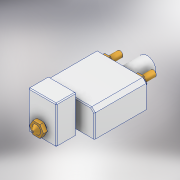
# Autodesk Inventor part: Arethusa
Saved by Autodesk Inventor 2022.1 (Build 261234020, 234B)
## iProperties
Created: 2022-04-17
Part Number: Arethusa
Material: Aluminum 6061
Document SubType Name: Modeling
Designer: Remo
Density: 2.7 g/cm^3
Appearance: Aluminum - Flat
Author: Remo
Autodesk Inventor part; units mm, degrees
ref_plane "YZ Plane" through (0, 0, 0) normal (1, 0, 0) x (0, 1, 0)
ref_plane "XZ Plane" through (0, 0, 0) normal (0, 1, 0) x (-1, 0, 0)
ref_plane "XY Plane" through (0, 0, 0) normal (0, 0, 1) x (1, 0, 0)
sketch "Sketch1" plane through (0, 0, 0) normal (0, 0, 1) x (1, 0, 0)
  line L0 (15, -7.5) -> (-15, -7.5)
  line L1 (-15, -7.5) -> (-15, 7.5)
  line L2 (-15, 7.5) -> (15, 7.5)
  line L3 (15, 7.5) -> (15, -7.5)
  line L4 (15, -7.5) -> (-15, 7.5) construction
  line L5 (-15, -7.5) -> (15, 7.5) construction
  point P0 (0, 0)
  dimension "d0" = 15
  dimension "d1" = 30
  constraints: 12 end point, 2 midpoint, 2 parallel, 1 horizontal, 1 perpendicular
  measures "d0" distance of L0.end L1.end
  measures "d1" distance of L1.end L2.end
extrude "Extrusion1" add sketch "Sketch1" along normal blind 30
sketch "Sketch2" plane through (0, 0, 30) normal (0, 0, 1) x (1, 0, 0)
  line L0 (15, 7.5) -> (-15, 7.5) projected
  line L1 (-15, 7.5) -> (-15, -7.5) projected
  line L2 (-15, -7.5) -> (15, -7.5) projected
  line L3 (15, -7.5) -> (15, 7.5) projected
  circle A0 centre (0, -1) radius 2.5
  point P0 (0, 0)
  dimension "d4" = 6.5
  dimension "d5" = 5
  constraints: 1 centre point, 1 vertical alignment
  measures "d4" distance from line of L2 A0.centre
  measures "d5" diameter of A0
extrude "Extrusion2" add sketch "Sketch2" along normal blind 3.3 contours A0
sketch "Sketch3" plane through (0, -1, 33.3) normal (0, 0, 1) x (1, 0, 0)
  circle A0 centre (0, 0) radius 2.5 projected
  line L0 (-8, 15) -> (8, 15)
  line L1 (8, 15) -> (8, -8)
  line L2 (8, -8) -> (-8, -8)
  line L3 (-8, -8) -> (-8, 15)
  line L4 (-8, 15) -> (8, -8) construction
  line L5 (8, 15) -> (-8, -8) construction
  line L6 (-15, -6.5) -> (15, -6.5) projected
  point P0 (0, 1)
  point P1 (0, 3.5)
  point P2 (0, 3.5)
  point P3 (-8, -6.5)
  point P4 (8, -6.5)
  dimension "d9" = 23
  dimension "d10" = 16
  dimension "d11" = 8
  constraints: 12 end point, 3 midpoint, 2 parallel, 1 horizontal, 1 perpendicular, 1 vertical alignment
  measures "d9" distance of L2.end L0.start
  measures "d10" distance of L0.start L0.end
  measures "d11" distance from line of L2 A0.centre
extrude "Extrusion3" add sketch "Sketch3" along normal blind 11.5 contours A0 | L0 L1 L6 L3
sketch "Sketch4" plane through (-15, -7.5, 0) normal (0, -1, 0) x (1, 0, 0)
  line L0 (0, 0) -> (30, 0) projected
  line L1 (30, 0) -> (30, 30) projected
  line L2 (0, 30) -> (30, 30) projected
  line L3 (0, 0) -> (0, 30) projected
  circle A0 centre (7, 7) radius 1.4
  circle A1 centre (23, 7) radius 1.4
  circle A2 centre (7, 23) radius 1.4
  circle A3 centre (23, 23) radius 1.4
  point P0 (15, 0)
  point P1 (15, 30)
  dimension "d16" = 16
  dimension "d19" = 16
  dimension "d22" = 8
  dimension "d23" = 7
  dimension "d24" = 2.8
  constraints: 4 centre point, 1 horizontal, 1 midpoint, 1 vertical, 6 other
  measures "d16" distance of A0.centre A1.centre
  measures "d19" distance of A0.centre A2.centre
  measures "d22" horizontal distance of A2.centre point (15, 30)
  measures "d23" distance from line of L0 A0.centre
  measures "d24" diameter of A2
extrude "Extrusion4" cut sketch "Sketch4" against normal blind 7 contours A0 | A1 | A2 | A3
sketch "Sketch5" plane through (0, -1, 44.8) normal (0, 0, 1) x (1, 0, 0)
  circle A0 centre (0, 0) radius 2.5 projected
  line L0 (-2.0207, 3.5) -> (2.0207, 3.5)
  line L1 (2.0207, 3.5) -> (4.0415, 0)
  line L2 (4.0415, 0) -> (2.0207, -3.5)
  line L3 (2.0207, -3.5) -> (-2.0207, -3.5)
  line L4 (-2.0207, -3.5) -> (-4.0415, 0)
  line L5 (-4.0415, 0) -> (-2.0207, 3.5)
  point P0 (0, 1)
  dimension "d35" = 7
  constraints: 12 end point, 1 coincident, 1 horizontal, 13 other
  measures "d35" distance between parallel lines of L3 L0
extrude "Extrusion5" add sketch "Sketch5" along normal blind 3.3 contours A0 | L0 L1 L2 L3 L4 L5
sketch "Sketch6" plane through (0, -1, 48.1) normal (0, 0, 1) x (1, 0, 0)
  line L0 (-4.0415, 0) -> (-2.0207, -3.5) projected
  line L1 (-2.0207, -3.5) -> (2.0207, -3.5) projected
  line L2 (2.0207, -3.5) -> (4.0415, 0) projected
  line L3 (4.0415, 0) -> (2.0207, 3.5) projected
  line L4 (2.0207, 3.5) -> (-2.0207, 3.5) projected
  line L5 (-2.0207, 3.5) -> (-4.0415, 0) projected
  circle A0 centre (0, 0) radius 2.5 projected
  point P0 (0, 1)
extrude "Extrusion6" add sketch "Sketch6" along normal blind 2 contours A0
chamfer "Chamfer1" distance 2 angle 45 1 edges at (-2.5, -1, 50.1)
sketch "Sketch7" plane through (0, -1, 44.8) normal (0, 0, 1) x (1, 0, 0)
  circle A0 centre (0, 0) radius 2.5 projected
  circle A1 centre (0, 0) radius 2.5 projected
  line L0 (-4.0415, 0) -> (-2.0207, -3.5) projected
  line L1 (-2.0207, -3.5) -> (2.0207, -3.5) projected
  line L2 (2.0207, -3.5) -> (4.0415, 0) projected
  line L3 (4.0415, 0) -> (2.0207, 3.5) projected
  line L4 (2.0207, 3.5) -> (-2.0207, 3.5) projected
  line L5 (-2.0207, 3.5) -> (-4.0415, 0) projected
  point P0 (0, 1)
extrude "Extrusion7" cut sketch "Sketch7" along normal blind 1
chamfer "Chamfer2" distance 2 angle 45 2 edges at (-15, 7.5, 15) (15, 7.5, 15)
chamfer "Chamfer3" distance 0.5 angle 45 22 edges at (-8, 3.25, 33.3) (8, 3.25, 33.3) (0, 14, 33.3) (8, 14, 39.05) (-8, 14, 39.05) (0, 14, 44.8) (-8, 3.25, 44.8) (-8, -7.5, 39.05) (0, -7.5, 33.3) (8, -7.5, 39.05) (0, -7.5, 44.8) (8, 3.25, 44.8) (0, 7.5, 30) (15, -1, 30) (14, 6.5, 30) (-15, -1, 30) (-14, 6.5, 30) (-15, -1, 0) (-14, 6.5, 0) (0, 7.5, 0) (14, 6.5, 0) (15, -1, 0)
sketch "Sketch8" plane through (0, 0, 0) normal (0, 0, -1) x (-1, 0, 0)
  line L0 (-14.5, -7.5) -> (-14.5, 5.2929) projected
  line L1 (14.5, -7.5) -> (-14.5, -7.5) projected
  line L2 (14.5, 5.2929) -> (14.5, -7.5) projected
  line L3 (12.7929, 7) -> (14.5, 5.2929) projected
  line L4 (-12.7929, 7) -> (12.7929, 7) projected
  line L5 (-14.5, 5.2929) -> (-12.7929, 7) projected
  line L6 (7.7679, 6) -> (11.2321, 6)
  line L7 (11.2321, 6) -> (12.9641, 3)
  line L8 (12.9641, 3) -> (11.2321, 0)
  line L9 (11.2321, 0) -> (7.7679, 0)
  line L10 (7.7679, 0) -> (6.0359, 3)
  line L11 (6.0359, 3) -> (7.7679, 6)
  line L12 (-11.2321, 6) -> (-7.7679, 6)
  line L13 (-7.7679, 6) -> (-6.0359, 3)
  line L14 (-6.0359, 3) -> (-7.7679, 0)
  line L15 (-7.7679, 0) -> (-11.2321, 0)
  line L16 (-11.2321, 0) -> (-12.9641, 3)
  line L17 (-12.9641, 3) -> (-11.2321, 6)
  point P0 (0, 0)
  point P1 (9.5, 3)
  point P2 (-9.5, 3)
  dimension "d51" = 6
  dimension "d52" = 5
  dimension "d53" = 5
  dimension "d54" = 4
  constraints: 24 end point, 2 horizontal, 1 collinear, 1 horizontal alignment, 26 other
  measures "d51" distance between parallel lines of L9 L6
  measures "d52" distance from line of L2 point (9.5, 3)
  measures "d53" distance from line of L0 point (-9.5, 3)
  measures "d54" distance from line of L4 point (9.5, 3)
extrude "Extrusion8" add sketch "Sketch8" along normal blind 2 contours L6 L7 L8 L9 L10 L11 | L12 L13 L14 L15 L16 L17
sketch "Sketch9" plane through (0, 0, -2) normal (0, 0, -1) x (-1, 0, 0)
  line L0 (6.0359, 3) -> (7.7679, 0) projected
  line L1 (7.7679, 0) -> (11.2321, 0) projected
  line L2 (11.2321, 0) -> (12.9641, 3) projected
  line L3 (12.9641, 3) -> (11.2321, 6) projected
  line L4 (11.2321, 6) -> (7.7679, 6) projected
  line L5 (7.7679, 6) -> (6.0359, 3) projected
  line L6 (-12.9641, 3) -> (-11.2321, 0) projected
  line L7 (-11.2321, 0) -> (-7.7679, 0) projected
  line L8 (-7.7679, 0) -> (-6.0359, 3) projected
  line L9 (-6.0359, 3) -> (-7.7679, 6) projected
  line L10 (-7.7679, 6) -> (-11.2321, 6) projected
  line L11 (-11.2321, 6) -> (-12.9641, 3) projected
  circle A0 centre (9.5, 3) radius 1.75
  circle A1 centre (-9.5, 3) radius 1.75
  circle A2 centre (9.5, 3) radius 1
  circle A3 centre (-9.5, 3) radius 1
  point P0 (0, 0)
  point P1 (9.5, 0)
  point P2 (-9.5, 0)
  dimension "d57" = 3.5
  dimension "d58" = 2
  constraints: 4 centre point, 2 coincident, 2 equal radius, 2 horizontal alignment, 2 midpoint, 2 vertical alignment
  measures "d57" diameter of A0
  measures "d58" diameter of A2
extrude "Extrusion9" add sketch "Sketch9" along normal blind 7 contours A0 | A1
sketch "Sketch10" plane through (0, 0, 0) normal (0, 0, -1) x (-1, 0, 0)
  line L0 (-12.9641, 3) -> (-11.2321, 6) projected
  line L1 (-11.2321, 6) -> (-7.7679, 6) projected
  line L2 (-7.7679, 6) -> (-6.0359, 3) projected
  line L3 (-6.0359, 3) -> (-7.7679, 0) projected
  line L4 (-7.7679, 0) -> (-11.2321, 0) projected
  line L5 (-11.2321, 0) -> (-12.9641, 3) projected
  line L6 (6.0359, 3) -> (7.7679, 6) projected
  line L7 (7.7679, 6) -> (11.2321, 6) projected
  line L8 (11.2321, 6) -> (12.9641, 3) projected
  line L9 (12.9641, 3) -> (11.2321, 0) projected
  line L10 (11.2321, 0) -> (7.7679, 0) projected
  line L11 (7.7679, 0) -> (6.0359, 3) projected
  line L12 (-14.5, -7.5) -> (-14.5, 5.2929) projected
  line L13 (14.5, -7.5) -> (-14.5, -7.5) projected
  line L14 (14.5, 5.2929) -> (14.5, -7.5) projected
  line L15 (12.7929, 7) -> (14.5, 5.2929) projected
  line L16 (-12.7929, 7) -> (12.7929, 7) projected
  line L17 (-14.5, 5.2929) -> (-12.7929, 7) projected
  circle A0 centre (0, -1) radius 2.5 projected
  circle A1 centre (0, -1) radius 0.5 projected
  circle A2 centre (0, -1) radius 5
  point P0 (0, 0)
  dimension "d61" = 10
  constraints: 1 centre point, 1 coincident
  measures "d61" diameter of A2
extrude "Extrusion10" add sketch "Sketch10" along normal blind 15 contours A0 | A1 | A2
equation "\"d22\" = 0.5 * d16"
equation "\"d53\" = d52"
body "Solid1"
